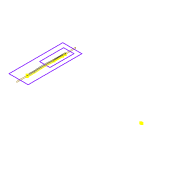
# Autodesk Inventor part: Part_11
Saved by Autodesk Inventor 2022 (Build 260153000, 153)
## iProperties
Created: 2022-04-26
Part Number: Part_11
Material: Generic
Document SubType Name: Modeling
Designer: dell
Density: 1 g/cm^3
Appearance: Default
Author: dell
Autodesk Inventor part; units mm, degrees
ref_plane "XZ Plane" through (0, 0, 0) normal (0, 1, 0) x (-1, 0, 0)
ref_plane "XY Plane" through (0, 0, 0) normal (0, 0, 1) x (1, 0, 0)
sketch "Sketch1" plane through (0, 0, 0) normal (0, 1, 0) x (-1, 0, 0)
  line L0 (0, 0) -> (0, -270.69) construction
  line L1 (-4, 0) -> (-4, -270.69)
  line L2 (4, -270.69) -> (4, 0)
  arc A0 (4, 0) -> (-4, 0) centre (0, 0) ccw
  arc A1 (-4, -270.69) -> (4, -270.69) centre (0, -270.69) ccw
  circle A2 centre (0, 0) radius 1.5
  circle A3 centre (0, -270.69) radius 1.5
  line L3 (0, -251.19) -> (0, -190.69) construction
  line L4 (1.5, -251.19) -> (1.5, -190.69)
  line L5 (-1.5, -190.69) -> (-1.5, -251.19)
  arc A4 (-1.5, -251.19) -> (1.5, -251.19) centre (0, -251.19) ccw
  arc A5 (1.5, -190.69) -> (-1.5, -190.69) centre (0, -190.69) ccw
  arc A6 (-4, -185.69) -> (-4, -50.69) centre (-700.7379, -118.19) ccw
  arc A7 (4, -185.69) -> (4, -50.69) centre (-692.7379, -118.19) ccw
  point P0 (0, -135.345)
  point P1 (0, -220.94)
  dimension "d0" = 270.69
  dimension "d1" = 8
  dimension "d2" = 3
  dimension "d3" = 3
  dimension "d10" = 3
  dimension "d11" = 19.5
  dimension "d12" = 80
  dimension "d13" = 85
  dimension "d14" = 220
  dimension "d15" = 700
  dimension "d16" = 700
  constraints: 16 end point, 12 point on circle, 8 centre point, 8 tangent, 6 point on line, 2 coincident, 2 horizontal alignment, 2 midpoint, 2 parallel, 1 vertical
  measures "d0" distance of L0.start L0.end
  measures "d1" diameter of A1
  measures "d2" diameter of A2
  measures "d3" diameter of A3
  measures "d10" diameter of A5
  measures "d11" distance of L0.end L3.start
  measures "d12" distance of L0.end L3.end
  measures "d13" vertical distance of A3.centre A6.start
  measures "d14" vertical distance of L0.end A6.end
  measures "d15" radius of A6
  measures "d16" radius of A7
extrude "Extrusion1" add sketch "Sketch1" along normal blind 8 contours A0 L2 A1 L1 A6 | A7 L2
sketch "Sketch2" plane through (0, 0, 0) normal (0, -1, 0) x (1, 0, 0)
  line L0 (4, 0) -> (4, -50.69) projected
  arc A0 (4, 0) -> (-4, 0) centre (0, 0) ccw projected
  line L1 (-4, -50.69) -> (-4, 0) projected
  arc A1 (-4, -50.69) -> (-4, -185.69) centre (692.7379, -118.19) ccw projected
  line L2 (-4, -270.69) -> (-4, -185.69) projected
  arc A2 (-4, -270.69) -> (4, -270.69) centre (0, -270.69) ccw projected
  line L3 (4, -185.69) -> (4, -270.69) projected
  arc A3 (4, -50.69) -> (4, -185.69) centre (700.7379, -118.19) ccw projected
  circle A4 centre (0, 0) radius 1.5 projected
  circle A5 centre (0, -270.69) radius 1.5 projected
  arc A6 (-1.5, -251.19) -> (1.5, -251.19) centre (0, -251.19) ccw projected
  line L4 (-1.5, -190.69) -> (-1.5, -251.19) projected
  arc A7 (1.5, -190.69) -> (-1.5, -190.69) centre (0, -190.69) ccw projected
  line L5 (1.5, -251.19) -> (1.5, -190.69) projected
sketch "Sketch3" plane through (0, 8, 0) normal (0, 1, 0) x (1, 0, 0)
  line L0 (-41.336, 299.9474) -> (32.3712, 299.9474)
  line L1 (32.3712, 299.9474) -> (32.3712, 128.1205)
  line L2 (32.3712, 128.1205) -> (-41.336, 128.1205)
  line L3 (-41.336, 128.1205) -> (-41.336, 299.9474)
  line L4 (-75.6075, 328.1158) -> (61.009, 328.1158)
  line L5 (61.009, 328.1158) -> (61.009, -56.3822)
  line L6 (61.009, -56.3822) -> (-75.6075, -56.3822)
  line L7 (-75.6075, -56.3822) -> (-75.6075, 328.1158)
  point P0 (0, 0)
  constraints: 16 end point, 4 parallel, 2 horizontal, 2 perpendicular
body "Solid1"
